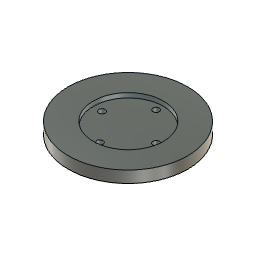
flowerbase (Autodesk Fusion 360 design; units mm, degrees)
Autodesk Fusion 360 part; units mm, degrees
sketch "Sketch1" plane through (0, 0, 0) normal (0, 0, 1) x (1, 0, 0)
  circle A0 centre (0, 0) radius 65
  dimension "d1" = 130
  constraint coincident A0.centre origin
  measures "d1" diameter of A0
extrude "Extrude1" add sketch "Sketch1" along normal blind 12.7
hole "Hole1" at (0.1314, 0.2629, 12.7) direction (0, 0, -1) diameter 76.2 depth 5 tip angle 180
hole "Hole2" at (-28.552, 0.2545, 7.7) direction (0, 0, -1) diameter 7 depth 7.7 tip angle 180
hole "Hole3" at (-0.3573, -30.3398, 7.7) direction (0, 0, -1) diameter 7 depth 7.7 tip angle 180
hole "Hole4" at (-0.4431, 30.9664, 7.7) direction (0, 0, -1) diameter 7 depth 7.7 tip angle 180
hole "Hole5" at (30.8296, -0.3123, 7.7) direction (0, 0, -1) diameter 7 depth 7.7 tip angle 180
sketch "Sketch2" plane through (0, 0, 0) normal (0, 0, 1) x (1, 0, 0)
sketch "Sketch3" plane through (0, 0, 12.7) normal (0, 0, 1) x (-1, 0, 0)
  circle A0 centre (-0.1314, -0.2629) radius 38.1
  circle A1 centre (0, 0) radius 65
